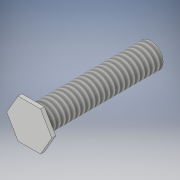
# Autodesk Inventor part: Pedal Bolt Outside Right
Saved by Autodesk Inventor 2019 (Build 230136000, 136)
## iProperties
Created: 2020-06-01
Part Number: Pedal Bolt Outside Right
Material: Generic
Document SubType Name: Modeling
Designer: 18186
Density: 1 g/cm^3
Appearance: Default
Author: 18186
Autodesk Inventor part; units mm, degrees
ref_plane "YZ Plane" through (0, 0, 0) normal (1, 0, 0) x (0, 1, 0)
ref_plane "XZ Plane" through (0, 0, 0) normal (0, 1, 0) x (-1, 0, 0)
ref_plane "XY Plane" through (0, 0, 0) normal (0, 0, 1) x (1, 0, 0)
sketch "Sketch1" plane through (0, 0, 0) normal (0, 0, 1) x (1, 0, 0)
  circle A0 centre (0, 0) radius 3.175
  dimension "d0" = 6.35
  constraints: 1 centre point, 1 coincident
  measures "d0" diameter of A0
extrude "Extrusion1" add sketch "Sketch1" along normal blind 30.148
sketch "Sketch2" plane through (0, 0, 30.148) normal (0, 0, 1) x (1, 0, 0)
  line L0 (5.7808, 0) -> (2.8904, -5.0064)
  line L1 (2.8904, -5.0064) -> (-2.8904, -5.0064)
  line L2 (-2.8904, -5.0064) -> (-5.7808, 0)
  line L3 (-5.7808, 0) -> (-2.8904, 5.0064)
  line L4 (-2.8904, 5.0064) -> (2.8904, 5.0064)
  line L5 (2.8904, 5.0064) -> (5.7808, 0)
  point P0 (0, 0)
  point P1 (0, 0)
  constraints: 12 end point, 1 coincident, 13 other
extrude "Extrusion2" add sketch "Sketch2" along normal blind 1
thread "Thread1" size "1/4-20 UNC" class "2A" standard "ANSI Unified Screw Threads" full length
body "Solid1"
